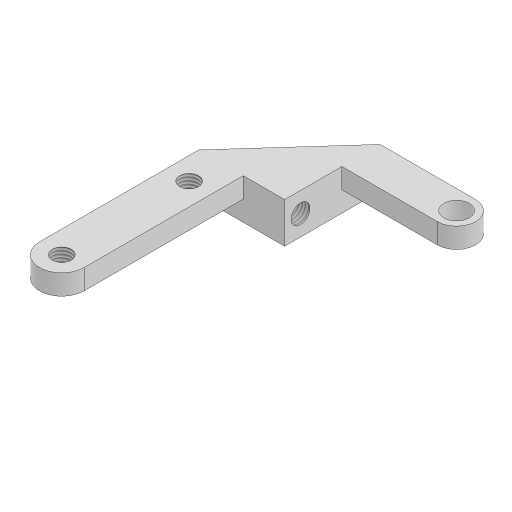
# Autodesk Inventor part: mgn9SlideBearingHolderWithCableManegment
Saved by Autodesk Inventor 2023 (Build 270158000, 158)
## iProperties
Created: 2022-11-03
Part Number: mgn9SlideBearingHolderWithCableManegment
Material: Generic
Document SubType Name: Modeling
Designer: deli
Density: 1 g/cm^3
Appearance: Default
Author: deli
Autodesk Inventor part; units mm, degrees
ref_plane "YZ Plane" through (0, 0, 0) normal (1, 0, 0) x (0, 1, 0)
ref_plane "XZ Plane" through (0, 0, 0) normal (0, 1, 0) x (-1, 0, 0)
ref_plane "XY Plane" through (0, 0, 0) normal (0, 0, 1) x (1, 0, 0)
sketch "Sketch1" plane through (0, 0, 0) normal (0, 1, 0) x (-1, 0, 0)
  circle A0 centre (16.4161, 48.6619) radius 1.5
  circle A1 centre (16.4161, 28.6619) radius 1.5
  arc A2 (19.9161, 48.6619) -> (12.9161, 48.6619) centre (16.4161, 48.6619) ccw
  line L0 (19.9161, 48.6619) -> (19.9161, 23.6619)
  line L1 (12.9161, 23.6619) -> (12.9161, 48.6619)
  line L2 (6.4161, 14.6619) -> (6.4161, 23.6619)
  line L3 (6.4161, 23.6619) -> (12.9161, 23.6619)
  line L4 (19.9161, 23.6619) -> (6.4161, 8.6619)
  line L5 (6.4161, 8.6619) -> (-8.5839, 8.6619)
  line L6 (-8.5839, 14.6619) -> (6.4161, 14.6619)
  arc A3 (-8.5839, 14.6619) -> (-8.5839, 8.6619) centre (-8.5839, 11.6619) ccw
  circle A4 centre (-8.5839, 11.6619) radius 2
  point P0 (0, 0)
  dimension "d0" = 3
  dimension "d1" = 2
  dimension "d2" = 20
  dimension "d20" = 10
  dimension "d27" = 3.5
  dimension "d35" = 5
  dimension "d36" = 9
  dimension "d38" = 15
  dimension "d39" = 6
  dimension "d40" = 4
  constraints: 14 end point, 5 centre point, 4 point on circle, 4 tangent, 2 coincident, 2 perpendicular, 2 point on line, 1 equal radius, 1 horizontal, 1 parallel, 1 vertical
  measures "d0" diameter of A0
  measures "d1" radial gap between concentric circles of A2 A0
  measures "d2" distance of A0.centre A1.centre
  measures "d20" distance from line of A1.centre L2
  measures "d27" distance from line of L0 A1.centre
  measures "d35" distance from line of L3 A1.centre
  measures "d36" distance of L2.start L2.end
  measures "d38" distance of L6.start L2.start
  measures "d39" diameter of A3
  measures "d40" diameter of A4
extrude "Extrusion1" add sketch "Sketch1" along normal blind 3.175
sketch "Sketch2" plane through (0, 3.175, 0) normal (0, 1, 0) x (1, 0, 0)
  line L0 (-12.9161, -48.6619) -> (-12.9161, -23.6619) projected
  line L1 (-12.9161, -23.6619) -> (-6.4161, -23.6619) projected
  line L2 (-6.4161, -23.6619) -> (-6.4161, -14.6619) projected
  line L3 (-6.4161, -14.6619) -> (8.5839, -14.6619) projected
  arc A0 (8.5839, -14.6619) -> (8.5839, -8.6619) centre (8.5839, -11.6619) ccw projected
  line L4 (8.5839, -8.6619) -> (-6.4161, -8.6619) projected
  line L5 (-6.4161, -8.6619) -> (-19.9161, -23.6619) projected
  line L6 (-19.9161, -23.6619) -> (-19.9161, -48.6619) projected
  arc A1 (-19.9161, -48.6619) -> (-12.9161, -48.6619) centre (-16.4161, -48.6619) ccw projected
  circle A2 centre (-16.4161, -48.6619) radius 1.5 projected
  circle A3 centre (-16.4161, -28.6619) radius 1.5 projected
  line L7 (-12.9161, -23.6619) -> (-19.9161, -23.6619)
  circle A4 centre (8.5839, -11.6619) radius 2 projected
  line L8 (-6.4161, -8.6619) -> (-6.4161, -14.6619)
  constraints: 4 end point, 1 collinear, 1 horizontal
extrude "Extrusion2" add sketch "Sketch2" against normal blind 6.35 contours L7 L5 L8 L2 L1
thread "Thread1" size "M3x0.5" class "6H" standard "ANSI Metric M Profile" full length
thread "Thread3" size "M3x0.5" class "6H" standard "ANSI Metric M Profile" full length
sketch "Sketch4" plane through (-6.4161, 0, 23.6619) normal (1, 0, 0) x (0, 0, 1)
  line L0 (0, 0) -> (25, 0) projected
  circle A0 centre (-2.5, 0) radius 1.5
  line L1 (0, 0) -> (0, 3.175) construction
  line L2 (0, -3.175) -> (25, -3.175) construction
  point P0 (-23.6619, 0)
  point P1 (-18.85, -3.175)
  dimension "d26" = 3
  dimension "d28" = 3.175
  dimension "d29" = 1
  constraints: 1 centre point, 1 coincident
  measures "d26" diameter of A0
  measures "d28" distance from line of L2 A0.centre
  measures "d29" distance edge to line of A0 L1
extrude "Extrusion4" cut sketch "Sketch4" against normal blind 8
thread "Thread4" size "M3x0.5" class "6H" standard "ANSI Metric M Profile" full length
equation "\"d27\" = d1 + 0.5 * d0"
body "Solid1"
